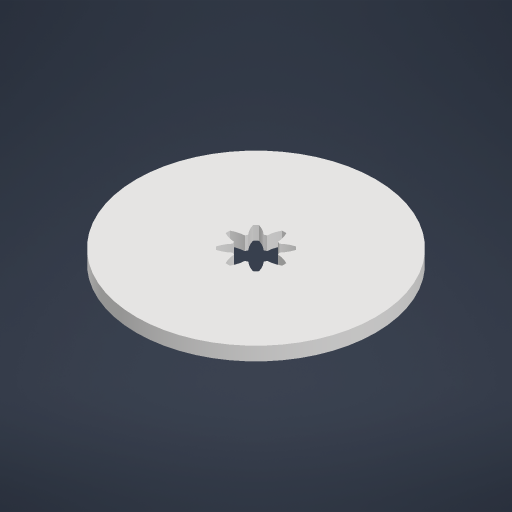
# Autodesk Inventor part: Part1
Saved by Autodesk Inventor 2023 (Build 270158000, 158)
## iProperties
Created: 2023-03-03
Part Number: Part1
Material: Generic
Document SubType Name: Modeling
Designer: Windows Macbook
Density: 1 g/cm^3
Appearance: Default
Author: Windows Macbook
Autodesk Inventor part; units mm, degrees
ref_plane "YZ Plane" through (0, 0, 0) normal (1, 0, 0) x (0, 1, 0)
ref_plane "XZ Plane" through (0, 0, 0) normal (0, 1, 0) x (-1, 0, 0)
ref_plane "XY Plane" through (0, 0, 0) normal (0, 0, 1) x (1, 0, 0)
sketch "Sketch1" plane through (0, 0, 0) normal (0, 1, 0) x (-1, 0, 0)
  circle A0 centre (0, -38.1) radius 13.97
  line L0 (0, -41.402) -> (0.254, -41.402) construction
  arc A1 (0.254, -41.3922) -> (0.635, -40.0302) centre (-2.4477, -39.9022) ccw
  arc A2 (-0.635, -40.0302) -> (-0.254, -41.3922) centre (2.6711, -39.8397) ccw
  arc A3 (-0.254, -41.3922) -> (0.254, -41.3922) centre (0, -38.1) ccw
  arc A4 (0.635, -40.0302) -> (0.7776, -39.9773) centre (0, -38.1) ccw
  arc A5 (-0.7776, -39.9773) -> (-0.635, -40.0302) centre (0, -38.1) ccw
  arc A6 (0.9159, -39.9139) -> (2.1483, -40.6076) centre (3.1189, -37.4414) ccw
  arc A7 (0.7776, -39.9773) -> (0.9159, -39.9139) centre (0, -38.1) ccw
  arc A8 (1.8139, -39.0159) -> (1.8773, -38.8776) centre (0, -38.1) ccw
  arc A9 (2.5076, -40.2483) -> (1.8139, -39.0159) centre (-0.4565, -41.1051) ccw
  arc A10 (2.1483, -40.6076) -> (2.5076, -40.2483) centre (0, -38.1) ccw
  arc A11 (1.9302, -38.735) -> (3.2922, -38.354) centre (1.7397, -35.4289) ccw
  arc A12 (1.8773, -38.8776) -> (1.9302, -38.735) centre (0, -38.1) ccw
  arc A13 (1.9302, -37.465) -> (1.8773, -37.3224) centre (0, -38.1) ccw
  arc A14 (3.2922, -37.846) -> (1.9302, -37.465) centre (1.8022, -40.5477) ccw
  arc A15 (3.2922, -38.354) -> (3.2922, -37.846) centre (0, -38.1) ccw
  arc A16 (1.8139, -37.1841) -> (2.5076, -35.9517) centre (-0.6586, -34.9811) ccw
  arc A17 (1.8773, -37.3224) -> (1.8139, -37.1841) centre (0, -38.1) ccw
  arc A18 (0.9159, -36.2861) -> (0.7776, -36.2227) centre (0, -38.1) ccw
  arc A19 (2.1483, -35.5924) -> (0.9159, -36.2861) centre (3.0051, -38.5565) ccw
  arc A20 (2.5076, -35.9517) -> (2.1483, -35.5924) centre (0, -38.1) ccw
  arc A21 (0.635, -36.1698) -> (0.254, -34.8078) centre (-2.6711, -36.3603) ccw
  arc A22 (0.7776, -36.2227) -> (0.635, -36.1698) centre (0, -38.1) ccw
  arc A23 (-0.635, -36.1698) -> (-0.7776, -36.2227) centre (0, -38.1) ccw
  arc A24 (-0.254, -34.8078) -> (-0.635, -36.1698) centre (2.4477, -36.2978) ccw
  arc A25 (0.254, -34.8078) -> (-0.254, -34.8078) centre (0, -38.1) ccw
  arc A26 (-0.9159, -36.2861) -> (-2.1483, -35.5924) centre (-3.1189, -38.7586) ccw
  arc A27 (-0.7776, -36.2227) -> (-0.9159, -36.2861) centre (0, -38.1) ccw
  arc A28 (-1.8139, -37.1841) -> (-1.8773, -37.3224) centre (0, -38.1) ccw
  arc A29 (-2.5076, -35.9517) -> (-1.8139, -37.1841) centre (0.4565, -35.0949) ccw
  arc A30 (-2.1483, -35.5924) -> (-2.5076, -35.9517) centre (0, -38.1) ccw
  arc A31 (-1.9302, -37.465) -> (-3.2922, -37.846) centre (-1.7397, -40.7711) ccw
  arc A32 (-1.8773, -37.3224) -> (-1.9302, -37.465) centre (0, -38.1) ccw
  arc A33 (-1.9302, -38.735) -> (-1.8773, -38.8776) centre (0, -38.1) ccw
  arc A34 (-3.2922, -38.354) -> (-1.9302, -38.735) centre (-1.8022, -35.6523) ccw
  arc A35 (-3.2922, -37.846) -> (-3.2922, -38.354) centre (0, -38.1) ccw
  arc A36 (-1.8139, -39.0159) -> (-2.5076, -40.2483) centre (0.6586, -41.2189) ccw
  arc A37 (-1.8773, -38.8776) -> (-1.8139, -39.0159) centre (0, -38.1) ccw
  arc A38 (-0.9159, -39.9139) -> (-0.7776, -39.9773) centre (0, -38.1) ccw
  arc A39 (-2.1483, -40.6076) -> (-0.9159, -39.9139) centre (-3.0051, -37.6435) ccw
  arc A40 (-2.5076, -40.2483) -> (-2.1483, -40.6076) centre (0, -38.1) ccw
  circle A41 centre (0, -48.26) radius 2.032
  circle A42 centre (0, -27.94) radius 2.032
  point P0 (0, 0)
  point P1 (2.3349, -40.4349)
  point P2 (3.302, -38.1)
  point P3 (2.3349, -35.7651)
  point P4 (0, -34.798)
  point P5 (-2.3349, -35.7651)
  point P6 (-3.302, -38.1)
  point P7 (-2.3349, -40.4349)
  point P8 (-0.7776, -39.9773)
  point P9 (-1.8773, -38.8776)
  point P10 (-1.8773, -37.3224)
  point P11 (-0.7776, -36.2227)
  point P12 (0.7776, -36.2227)
  point P13 (1.8773, -37.3224)
  point P14 (1.8773, -38.8776)
  point P15 (0.7776, -39.9773)
  dimension "d39" = 360
  dimension "d44" = 4.064
  dimension "d46" = 4.064
  constraints: 88 point on circle, 43 centre point, 2 coincident, 2 end point, 1 horizontal, 129 other
  measures "d44" diameter of A41
  measures "d46" diameter of A42
extrude "Extrusion1" add sketch "Sketch1" along normal blind 1.5875 contours A0 | A41 | A42
body "Solid1"
